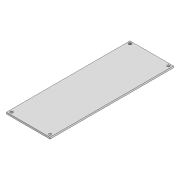
# Autodesk Inventor part: Cover
Saved by Autodesk Inventor 2022 (Build 260153000, 153)
## iProperties
Created: 2021-11-16
Part Number: Cover
Material: Generic
Document SubType Name: Modeling
Designer: Vking
Density: 1 g/cm^3
Appearance: Default
Author: Vking
Autodesk Inventor part; units mm, degrees
ref_plane "YZ Plane" through (0, 0, 0) normal (1, 0, 0) x (0, 1, 0)
ref_plane "XZ Plane" through (0, 0, 0) normal (0, 1, 0) x (-1, 0, 0)
ref_plane "XY Plane" through (0, 0, 0) normal (0, 0, 1) x (1, 0, 0)
sketch "Sketch1" plane through (0, 0, 0) normal (0, 1, 0) x (-1, 0, 0)
  line L0 (28.7334, 91.142) -> (-21.2666, 91.142)
  line L1 (-21.2666, 91.142) -> (-21.2666, -78.858)
  line L2 (-21.2666, -78.858) -> (28.7334, -78.858)
  line L3 (28.7334, -78.858) -> (28.7334, 91.142)
  line L4 (36.3534, 98.762) -> (-28.8866, 98.762)
  line L5 (-28.8866, 98.762) -> (-28.8866, -86.478)
  line L6 (-28.8866, -86.478) -> (36.3534, -86.478)
  line L7 (36.3534, -86.478) -> (36.3534, 98.762)
  circle A0 centre (32.5434, 94.952) radius 2
  circle A1 centre (-25.0766, 94.952) radius 2
  circle A2 centre (-25.0766, -82.668) radius 2
  circle A3 centre (32.5434, -82.668) radius 2
  dimension "d0" = 170
  dimension "d1" = 7.62
  dimension "d9" = 50
  dimension "d34" = 3.81
  dimension "d35" = 3.81
  dimension "d36" = 4
  dimension "d37" = 3.81
  dimension "d38" = 3.81
  dimension "d39" = 4
  dimension "d40" = 3.81
  dimension "d41" = 3.81
  dimension "d42" = 4
  dimension "d43" = 3.81
  dimension "d44" = 3.81
  dimension "d45" = 4
  dimension "d48" = 185.24
  constraints: 16 end point, 4 centre point, 4 parallel, 2 perpendicular, 1 horizontal, 3 other
  measures "d0" distance of L2.end L0.start
  measures "d1" distance between parallel lines of L3 L7
  measures "d9" distance of L1.end L2.end
  measures "d34" distance from line of L6 A3.centre
  measures "d35" distance from line of A3.centre L7
  measures "d36" diameter of A3
  measures "d37" distance from line of L7 A0.centre
  measures "d38" distance from line of L4 A0.centre
  measures "d39" diameter of A0
  measures "d40" distance from line of L4 A1.centre
  measures "d41" distance from line of L5 A1.centre
  measures "d42" diameter of A1
  measures "d43" distance from line of L5 A2.centre
  measures "d44" distance from line of A2.centre L6
  measures "d45" diameter of A2
  measures "d48" distance of L4.end L5.end
extrude "Extrusion1" add sketch "Sketch1" along normal blind 2.54 contours L3 L2 L1 L0 | L7 L6 L5 L4
body "Solid1"
